Autodesk Fusion 360 part; units mm, degrees
(part 3 of 3)
  spline S37 degree 5 poles (-0.4472, -23.7562) (-0.4505, -23.7623) (-0.4571, -23.7746) (-0.4669, -23.793) (-0.4799, -23.8176) (-0.496, -23.8484) (-0.512, -23.8792) (-0.5278, -23.91) (-0.5434, -23.9408) (-0.5589, -23.9717) (-0.5742, -24.0026) (-0.5894, -24.0336) (-0.6044, -24.0645) (-0.6192, -24.0955) (-0.6339, -24.1265) (-0.6484, -24.1575) (-0.6627, -24.1886) (-0.6769, -24.2197) (-0.6909, -24.2508) (-0.7047, -24.2819) (-0.7183, -24.3131) (-0.7318, -24.3442) (-0.7451, -24.3754) (-0.7583, -24.4066) (-0.7712, -24.4379) (-0.784, -24.4691) (-0.7966, -24.5004) (-0.809, -24.5317) (-0.8213, -24.563) (-0.8333, -24.5943) (-0.8452, -24.6257) (-0.8569, -24.657) (-0.8684, -24.6884) (-0.8797, -24.7198) (-0.8908, -24.7512) (-0.9017, -24.7826) (-0.9124, -24.8141) (-0.923, -24.8455) (-0.9333, -24.877) (-0.9434, -24.9085) (-0.9533, -24.94) (-0.963, -24.9715) (-0.9725, -25.003) (-0.9818, -25.0346) (-0.9909, -25.0661) (-0.9997, -25.0977) (-1.0083, -25.1292) (-1.0168, -25.1608) (-1.0249, -25.1924) (-1.0329, -25.224) (-1.0406, -25.2556) (-1.048, -25.2872) (-1.0552, -25.3188) (-1.0622, -25.3504) (-1.0688, -25.382) (-1.0752, -25.4136) (-1.0814, -25.4452) (-1.0873, -25.4768) (-1.093, -25.5084) (-1.0984, -25.5401) (-1.1035, -25.5717) (-1.1081, -25.6033) (-1.1123, -25.6349) (-1.1161, -25.6665) (-1.1196, -25.6981) (-1.1227, -25.7297) (-1.1257, -25.7612) (-1.1284, -25.7928) (-1.1308, -25.8243) (-1.1327, -25.8558) (-1.1337, -25.8873) (-1.1335, -25.9124) (-1.1327, -25.9313) (-1.1319, -25.9438) (-1.1314, -25.9501) knots -1 -1 -1 -1 -1 -1 -0.98571429 -0.97142857 -0.95714286 -0.94285714 -0.92857143 -0.91428571 -0.9 -0.88571429 -0.87142857 -0.85714286 -0.84285714 -0.82857143 -0.81428571 -0.8 -0.78571429 -0.77142857 -0.75714286 -0.74285714 -0.72857143 -0.71428571 -0.7 -0.68571429 -0.67142857 -0.65714286 -0.64285714 -0.62857143 -0.61428571 -0.6 -0.58571429 -0.57142857 -0.55714286 -0.54285714 -0.52857143 -0.51428571 -0.5 -0.48571429 -0.47142857 -0.45714286 -0.44285714 -0.42857143 -0.41428571 -0.4 -0.38571429 -0.37142857 -0.35714286 -0.34285714 -0.32857143 -0.31428571 -0.3 -0.28571429 -0.27142857 -0.25714286 -0.24285714 -0.22857143 -0.21428571 -0.2 -0.18571429 -0.17142857 -0.15714286 -0.14285714 -0.12857143 -0.11428571 -0.1 -0.08571429 -0.07142857 -0.05714286 -0.04285714 -0.02857143 -0.01428571 0 0 0 0 0 0
  line L37 (-1.1314, -25.9501) -> (-1.0999, -26.3476)
  arc A75 (-1.3245, -26.6162) -> (-1.0999, -26.3476) centre (-1.3491, -26.3674) ccw
  arc A76 (-1.3245, -26.6162) -> (-2.1846, -26.7294) centre (0, -40) ccw
  arc A77 (-2.4711, -26.5282) -> (-2.1846, -26.7294) centre (-2.2252, -26.4827) ccw
  line L38 (-2.4711, -26.5282) -> (-2.5435, -26.136)
  spline S38 degree 5 poles (-2.5435, -26.136) (-2.5447, -26.1298) (-2.5471, -26.1175) (-2.5512, -26.0991) (-2.5576, -26.0747) (-2.5667, -26.0446) (-2.5766, -26.0146) (-2.5871, -25.9848) (-2.5979, -25.9551) (-2.609, -25.9253) (-2.6202, -25.8956) (-2.6317, -25.866) (-2.6435, -25.8365) (-2.6558, -25.807) (-2.6685, -25.7777) (-2.6815, -25.7485) (-2.6949, -25.7193) (-2.7086, -25.6903) (-2.7225, -25.6613) (-2.7367, -25.6323) (-2.751, -25.6034) (-2.7656, -25.5746) (-2.7805, -25.5459) (-2.7956, -25.5172) (-2.811, -25.4886) (-2.8266, -25.4601) (-2.8425, -25.4317) (-2.8586, -25.4033) (-2.8749, -25.375) (-2.8914, -25.3467) (-2.9081, -25.3185) (-2.925, -25.2904) (-2.9421, -25.2623) (-2.9594, -25.2343) (-2.977, -25.2064) (-2.9947, -25.1786) (-3.0126, -25.1508) (-3.0307, -25.123) (-3.0491, -25.0954) (-3.0675, -25.0678) (-3.0862, -25.0403) (-3.1051, -25.0128) (-3.1241, -24.9854) (-3.1434, -24.958) (-3.1628, -24.9308) (-3.1823, -24.9036) (-3.2021, -24.8764) (-3.222, -24.8494) (-3.2421, -24.8223) (-3.2624, -24.7954) (-3.2828, -24.7685) (-3.3034, -24.7417) (-3.3242, -24.715) (-3.3451, -24.6883) (-3.3662, -24.6617) (-3.3875, -24.6351) (-3.4089, -24.6086) (-3.4304, -24.5822) (-3.4522, -24.5558) (-3.4741, -24.5296) (-3.4961, -24.5033) (-3.5183, -24.4772) (-3.5406, -24.4511) (-3.5631, -24.4251) (-3.5858, -24.3991) (-3.6086, -24.3732) (-3.6315, -24.3474) (-3.6546, -24.3216) (-3.6779, -24.296) (-3.7012, -24.2703) (-3.7248, -24.2448) (-3.7437, -24.2244) (-3.758, -24.2092) (-3.7675, -24.199) (-3.7723, -24.1939) knots 0 0 0 0 0 0 0.01428571 0.02857143 0.04285714 0.05714286 0.07142857 0.08571429 0.1 0.11428571 0.12857143 0.14285714 0.15714286 0.17142857 0.18571429 0.2 0.21428571 0.22857143 0.24285714 0.25714286 0.27142857 0.28571429 0.3 0.31428571 0.32857143 0.34285714 0.35714286 0.37142857 0.38571429 0.4 0.41428571 0.42857143 0.44285714 0.45714286 0.47142857 0.48571429 0.5 0.51428571 0.52857143 0.54285714 0.55714286 0.57142857 0.58571429 0.6 0.61428571 0.62857143 0.64285714 0.65714286 0.67142857 0.68571429 0.7 0.71428571 0.72857143 0.74285714 0.75714286 0.77142857 0.78571429 0.8 0.81428571 0.82857143 0.84285714 0.85714286 0.87142857 0.88571429 0.9 0.91428571 0.92857143 0.94285714 0.95714286 0.97142857 0.98571429 1 1 1 1 1 1
  arc A78 (-3.7723, -24.1939) -> (-4.6361, -24.4254) centre (0, -40) ccw
  spline S39 degree 5 poles (-4.6361, -24.4254) (-4.6377, -24.4322) (-4.6409, -24.4457) (-4.6457, -24.4661) (-4.6519, -24.4932) (-4.6595, -24.5271) (-4.6669, -24.561) (-4.6742, -24.5948) (-4.6813, -24.6287) (-4.6883, -24.6625) (-4.6951, -24.6963) (-4.7017, -24.7301) (-4.7082, -24.7639) (-4.7145, -24.7977) (-4.7206, -24.8314) (-4.7266, -24.8652) (-4.7324, -24.8989) (-4.738, -24.9326) (-4.7435, -24.9662) (-4.7488, -24.9999) (-4.754, -25.0335) (-4.7589, -25.0671) (-4.7637, -25.1007) (-4.7683, -25.1342) (-4.7727, -25.1677) (-4.777, -25.2012) (-4.7811, -25.2347) (-4.785, -25.2681) (-4.7887, -25.3016) (-4.7922, -25.3349) (-4.7956, -25.3683) (-4.7987, -25.4016) (-4.8017, -25.4349) (-4.8045, -25.4681) (-4.8071, -25.5014) (-4.8095, -25.5345) (-4.8118, -25.5677) (-4.8138, -25.6008) (-4.8156, -25.6339) (-4.8172, -25.6669) (-4.8187, -25.6999) (-4.8199, -25.7328) (-4.8209, -25.7658) (-4.8217, -25.7986) (-4.8223, -25.8314) (-4.8227, -25.8642) (-4.8228, -25.8969) (-4.8228, -25.9296) (-4.8225, -25.9622) (-4.822, -25.9948) (-4.8213, -26.0273) (-4.8203, -26.0597) (-4.8191, -26.0921) (-4.8176, -26.1244) (-4.8158, -26.1567) (-4.8138, -26.1889) (-4.8116, -26.221) (-4.8092, -26.2531) (-4.8065, -26.2851) (-4.8035, -26.3171) (-4.8002, -26.3489) (-4.7965, -26.3806) (-4.7924, -26.4123) (-4.7879, -26.4438) (-4.783, -26.4752) (-4.7779, -26.5065) (-4.7726, -26.5377) (-4.7671, -26.5689) (-4.7613, -26.6) (-4.7549, -26.6309) (-4.7477, -26.6616) (-4.741, -26.6858) (-4.7354, -26.7038) (-4.7313, -26.7157) (-4.7292, -26.7217) knots -1 -1 -1 -1 -1 -1 -0.98571429 -0.97142857 -0.95714286 -0.94285714 -0.92857143 -0.91428571 -0.9 -0.88571429 -0.87142857 -0.85714286 -0.84285714 -0.82857143 -0.81428571 -0.8 -0.78571429 -0.77142857 -0.75714286 -0.74285714 -0.72857143 -0.71428571 -0.7 -0.68571429 -0.67142857 -0.65714286 -0.64285714 -0.62857143 -0.61428571 -0.6 -0.58571429 -0.57142857 -0.55714286 -0.54285714 -0.52857143 -0.51428571 -0.5 -0.48571429 -0.47142857 -0.45714286 -0.44285714 -0.42857143 -0.41428571 -0.4 -0.38571429 -0.37142857 -0.35714286 -0.34285714 -0.32857143 -0.31428571 -0.3 -0.28571429 -0.27142857 -0.25714286 -0.24285714 -0.22857143 -0.21428571 -0.2 -0.18571429 -0.17142857 -0.15714286 -0.14285714 -0.12857143 -0.11428571 -0.1 -0.08571429 -0.07142857 -0.05714286 -0.04285714 -0.02857143 -0.01428571 0 0 0 0 0 0
  line L39 (-4.7292, -26.7217) -> (-4.5959, -27.0975)
  arc A79 (-4.7433, -27.415) -> (-4.5959, -27.0975) centre (-4.8315, -27.1811) ccw
  arc A80 (-4.7433, -27.415) -> (-5.5449, -27.747) centre (0, -40) ccw
  arc A81 (-5.8737, -27.6268) -> (-5.5449, -27.747) centre (-5.648, -27.5193) ccw
  line L40 (-5.8737, -27.6268) -> (-6.0451, -27.2667)
  spline S40 degree 5 poles (-6.0451, -27.2667) (-6.0478, -27.261) (-6.0534, -27.2497) (-6.0621, -27.233) (-6.0745, -27.2112) (-6.0911, -27.1844) (-6.1085, -27.1581) (-6.1264, -27.132) (-6.1445, -27.106) (-6.1629, -27.0802) (-6.1814, -27.0544) (-6.2002, -27.0287) (-6.2193, -27.0033) (-6.2387, -26.978) (-6.2585, -26.953) (-6.2787, -26.9281) (-6.2992, -26.9034) (-6.3199, -26.8789) (-6.3409, -26.8545) (-6.362, -26.8302) (-6.3834, -26.806) (-6.405, -26.782) (-6.4268, -26.7581) (-6.4488, -26.7343) (-6.471, -26.7106) (-6.4935, -26.6871) (-6.5162, -26.6638) (-6.5391, -26.6405) (-6.5621, -26.6174) (-6.5854, -26.5943) (-6.6088, -26.5714) (-6.6324, -26.5486) (-6.6562, -26.526) (-6.6802, -26.5034) (-6.7044, -26.481) (-6.7287, -26.4587) (-6.7532, -26.4365) (-6.7779, -26.4144) (-6.8028, -26.3924) (-6.8278, -26.3705) (-6.8529, -26.3488) (-6.8783, -26.3271) (-6.9038, -26.3056) (-6.9294, -26.2842) (-6.9552, -26.2628) (-6.9812, -26.2416) (-7.0073, -26.2205) (-7.0335, -26.1995) (-7.0599, -26.1786) (-7.0865, -26.1578) (-7.1132, -26.1372) (-7.14, -26.1166) (-7.167, -26.0961) (-7.1941, -26.0758) (-7.2214, -26.0555) (-7.2488, -26.0354) (-7.2763, -26.0153) (-7.304, -25.9954) (-7.3318, -25.9756) (-7.3597, -25.9558) (-7.3878, -25.9362) (-7.416, -25.9167) (-7.4443, -25.8973) (-7.4728, -25.878) (-7.5014, -25.8588) (-7.5301, -25.8397) (-7.559, -25.8207) (-7.5879, -25.8018) (-7.617, -25.783) (-7.6463, -25.7643) (-7.6756, -25.7457) (-7.6992, -25.7309) (-7.7169, -25.7198) (-7.7287, -25.7125) (-7.7347, -25.7088) knots 0 0 0 0 0 0 0.01428571 0.02857143 0.04285714 0.05714286 0.07142857 0.08571429 0.1 0.11428571 0.12857143 0.14285714 0.15714286 0.17142857 0.18571429 0.2 0.21428571 0.22857143 0.24285714 0.25714286 0.27142857 0.28571429 0.3 0.31428571 0.32857143 0.34285714 0.35714286 0.37142857 0.38571429 0.4 0.41428571 0.42857143 0.44285714 0.45714286 0.47142857 0.48571429 0.5 0.51428571 0.52857143 0.54285714 0.55714286 0.57142857 0.58571429 0.6 0.61428571 0.62857143 0.64285714 0.65714286 0.67142857 0.68571429 0.7 0.71428571 0.72857143 0.74285714 0.75714286 0.77142857 0.78571429 0.8 0.81428571 0.82857143 0.84285714 0.85714286 0.87142857 0.88571429 0.9 0.91428571 0.92857143 0.94285714 0.95714286 0.97142857 0.98571429 1 1 1 1 1 1
  arc A82 (-7.7347, -25.7088) -> (-8.5092, -26.156) centre (0, -40) ccw
  spline S41 degree 5 poles (-8.5092, -26.156) (-8.509, -26.163) (-8.5085, -26.1769) (-8.5078, -26.1978) (-8.5068, -26.2256) (-8.5054, -26.2603) (-8.5038, -26.2949) (-8.5021, -26.3295) (-8.5002, -26.3641) (-8.4982, -26.3986) (-8.496, -26.433) (-8.4936, -26.4673) (-8.4911, -26.5017) (-8.4885, -26.5359) (-8.4857, -26.5701) (-8.4827, -26.6042) (-8.4796, -26.6383) (-8.4763, -26.6723) (-8.4729, -26.7062) (-8.4693, -26.7401) (-8.4656, -26.7739) (-8.4617, -26.8076) (-8.4576, -26.8413) (-8.4534, -26.8749) (-8.449, -26.9084) (-8.4444, -26.9419) (-8.4397, -26.9752) (-8.4348, -27.0086) (-8.4298, -27.0418) (-8.4245, -27.075) (-8.4191, -27.108) (-8.4136, -27.141) (-8.4078, -27.174) (-8.4019, -27.2068) (-8.3958, -27.2396) (-8.3896, -27.2722) (-8.3832, -27.3048) (-8.3765, -27.3373) (-8.3697, -27.3698) (-8.3628, -27.4021) (-8.3556, -27.4343) (-8.3483, -27.4665) (-8.3407, -27.4985) (-8.333, -27.5305) (-8.3251, -27.5623) (-8.3169, -27.5941) (-8.3086, -27.6257) (-8.3001, -27.6572) (-8.2914, -27.6887) (-8.2825, -27.72) (-8.2734, -27.7512) (-8.2641, -27.7823) (-8.2545, -27.8133) (-8.2447, -27.8441) (-8.2346, -27.8748) (-8.2244, -27.9054) (-8.2139, -27.9359) (-8.2032, -27.9662) (-8.1924, -27.9965) (-8.1812, -28.0265) (-8.1698, -28.0564) (-8.158, -28.0861) (-8.1459, -28.1156) (-8.1334, -28.1449) (-8.1205, -28.174) (-8.1075, -28.2029) (-8.0943, -28.2317) (-8.0808, -28.2604) (-8.0672, -28.2889) (-8.0531, -28.3171) (-8.0382, -28.3449) (-8.0255, -28.3666) (-8.0154, -28.3825) (-8.0083, -28.3929) (-8.0048, -28.3981) knots -1 -1 -1 -1 -1 -1 -0.98571429 -0.97142857 -0.95714286 -0.94285714 -0.92857143 -0.91428571 -0.9 -0.88571429 -0.87142857 -0.85714286 -0.84285714 -0.82857143 -0.81428571 -0.8 -0.78571429 -0.77142857 -0.75714286 -0.74285714 -0.72857143 -0.71428571 -0.7 -0.68571429 -0.67142857 -0.65714286 -0.64285714 -0.62857143 -0.61428571 -0.6 -0.58571429 -0.57142857 -0.55714286 -0.54285714 -0.52857143 -0.51428571 -0.5 -0.48571429 -0.47142857 -0.45714286 -0.44285714 -0.42857143 -0.41428571 -0.4 -0.38571429 -0.37142857 -0.35714286 -0.34285714 -0.32857143 -0.31428571 -0.3 -0.28571429 -0.27142857 -0.25714286 -0.24285714 -0.22857143 -0.21428571 -0.2 -0.18571429 -0.17142857 -0.15714286 -0.14285714 -0.12857143 -0.11428571 -0.1 -0.08571429 -0.07142857 -0.05714286 -0.04285714 -0.02857143 -0.01428571 0 0 0 0 0 0
  line L41 (-8.0048, -28.3981) -> (-7.7787, -28.7266)
  arc A83 (-7.8389, -29.0715) -> (-7.7787, -28.7266) centre (-7.9847, -28.8684) ccw
  arc A84 (-7.8389, -29.0715) -> (-8.5272, -29.5997) centre (0, -40) ccw
  arc A85 (-8.876, -29.5686) -> (-8.5272, -29.5997) centre (-8.6858, -29.4063) ccw
  line L42 (-8.876, -29.5686) -> (-9.1348, -29.2652)
  spline S42 degree 5 poles (-9.1348, -29.2652) (-9.1388, -29.2604) (-9.1471, -29.2509) (-9.1599, -29.2371) (-9.1775, -29.2191) (-9.2005, -29.1976) (-9.2241, -29.1766) (-9.2481, -29.1561) (-9.2724, -29.1357) (-9.2968, -29.1155) (-9.3213, -29.0954) (-9.3461, -29.0755) (-9.3711, -29.0558) (-9.3965, -29.0364) (-9.4221, -29.0174) (-9.448, -28.9986) (-9.4742, -28.98) (-9.5006, -28.9617) (-9.5271, -28.9435) (-9.5539, -28.9256) (-9.5807, -28.9077) (-9.6078, -28.8901) (-9.635, -28.8726) (-9.6625, -28.8554) (-9.6901, -28.8383) (-9.7179, -28.8214) (-9.7458, -28.8047) (-9.7739, -28.7881) (-9.8022, -28.7718) (-9.8306, -28.7556) (-9.8592, -28.7395) (-9.8879, -28.7236) (-9.9168, -28.7079) (-9.9458, -28.6923) (-9.9749, -28.6769) (-10.0042, -28.6616) (-10.0336, -28.6465) (-10.0632, -28.6315) (-10.0929, -28.6167) (-10.1227, -28.6021) (-10.1526, -28.5876) (-10.1827, -28.5732) (-10.2129, -28.559) (-10.2432, -28.545) (-10.2736, -28.5311) (-10.3042, -28.5173) (-10.3349, -28.5037) (-10.3657, -28.4902) (-10.3966, -28.4768) (-10.4276, -28.4636) (-10.4588, -28.4506) (-10.49, -28.4376) (-10.5214, -28.4249) (-10.5528, -28.4122) (-10.5844, -28.3997) (-10.6161, -28.3873) (-10.6479, -28.3751) (-10.6798, -28.363) (-10.7118, -28.3511) (-10.7438, -28.3392) (-10.776, -28.3275) (-10.8083, -28.316) (-10.8407, -28.3046) (-10.8732, -28.2933) (-10.9058, -28.2821) (-10.9385, -28.2711) (-10.9713, -28.2602) (-11.0042, -28.2495) (-11.0371, -28.2388) (-11.0702, -28.2283) (-11.1033, -28.218) (-11.1299, -28.2098) (-11.1499, -28.2037) (-11.1633, -28.1997) (-11.1699, -28.1977) knots 0 0 0 0 0 0 0.01428571 0.02857143 0.04285714 0.05714286 0.07142857 0.08571429 0.1 0.11428571 0.12857143 0.14285714 0.15714286 0.17142857 0.18571429 0.2 0.21428571 0.22857143 0.24285714 0.25714286 0.27142857 0.28571429 0.3 0.31428571 0.32857143 0.34285714 0.35714286 0.37142857 0.38571429 0.4 0.41428571 0.42857143 0.44285714 0.45714286 0.47142857 0.48571429 0.5 0.51428571 0.52857143 0.54285714 0.55714286 0.57142857 0.58571429 0.6 0.61428571 0.62857143 0.64285714 0.65714286 0.67142857 0.68571429 0.7 0.71428571 0.72857143 0.74285714 0.75714286 0.77142857 0.78571429 0.8 0.81428571 0.82857143 0.84285714 0.85714286 0.87142857 0.88571429 0.9 0.91428571 0.92857143 0.94285714 0.95714286 0.97142857 0.98571429 1 1 1 1 1 1
  arc A86 (-11.1699, -28.1977) -> (-11.8023, -28.8301) centre (0, -40) ccw
  spline S43 degree 5 poles (-11.8023, -28.8301) (-11.8003, -28.8367) (-11.7963, -28.8501) (-11.7902, -28.8701) (-11.782, -28.8967) (-11.7717, -28.9298) (-11.7612, -28.9629) (-11.7505, -28.9958) (-11.7398, -29.0287) (-11.7289, -29.0615) (-11.7179, -29.0942) (-11.7067, -29.1268) (-11.6954, -29.1593) (-11.684, -29.1917) (-11.6725, -29.224) (-11.6608, -29.2562) (-11.6489, -29.2882) (-11.637, -29.3202) (-11.6249, -29.3521) (-11.6127, -29.3839) (-11.6003, -29.4156) (-11.5878, -29.4472) (-11.5751, -29.4786) (-11.5624, -29.51) (-11.5494, -29.5412) (-11.5364, -29.5724) (-11.5232, -29.6034) (-11.5098, -29.6343) (-11.4963, -29.6651) (-11.4827, -29.6958) (-11.4689, -29.7264) (-11.455, -29.7568) (-11.441, -29.7871) (-11.4268, -29.8173) (-11.4124, -29.8474) (-11.3979, -29.8773) (-11.3833, -29.9071) (-11.3685, -29.9368) (-11.3535, -29.9664) (-11.3384, -29.9958) (-11.3231, -30.0251) (-11.3077, -30.0542) (-11.2921, -30.0832) (-11.2764, -30.1121) (-11.2605, -30.1408) (-11.2444, -30.1694) (-11.2282, -30.1978) (-11.2119, -30.2261) (-11.1953, -30.2542) (-11.1786, -30.2821) (-11.1617, -30.3099) (-11.1446, -30.3375) (-11.1274, -30.365) (-11.1099, -30.3922) (-11.0923, -30.4193) (-11.0744, -30.4461) (-11.0565, -30.4729) (-11.0383, -30.4994) (-11.02, -30.5258) (-11.0014, -30.552) (-10.9826, -30.5779) (-10.9636, -30.6035) (-10.9442, -30.6289) (-10.9245, -30.6539) (-10.9046, -30.6787) (-10.8845, -30.7032) (-10.8643, -30.7276) (-10.8439, -30.7519) (-10.8234, -30.7759) (-10.8024, -30.7995) (-10.7809, -30.8225) (-10.7629, -30.8401) (-10.7491, -30.8529) (-10.7396, -30.8612) (-10.7348, -30.8652) knots -1 -1 -1 -1 -1 -1 -0.98571429 -0.97142857 -0.95714286 -0.94285714 -0.92857143 -0.91428571 -0.9 -0.88571429 -0.87142857 -0.85714286 -0.84285714 -0.82857143 -0.81428571 -0.8 -0.78571429 -0.77142857 -0.75714286 -0.74285714 -0.72857143 -0.71428571 -0.7 -0.68571429 -0.67142857 -0.65714286 -0.64285714 -0.62857143 -0.61428571 -0.6 -0.58571429 -0.57142857 -0.55714286 -0.54285714 -0.52857143 -0.51428571 -0.5 -0.48571429 -0.47142857 -0.45714286 -0.44285714 -0.42857143 -0.41428571 -0.4 -0.38571429 -0.37142857 -0.35714286 -0.34285714 -0.32857143 -0.31428571 -0.3 -0.28571429 -0.27142857 -0.25714286 -0.24285714 -0.22857143 -0.21428571 -0.2 -0.18571429 -0.17142857 -0.15714286 -0.14285714 -0.12857143 -0.11428571 -0.1 -0.08571429 -0.07142857 -0.05714286 -0.04285714 -0.02857143 -0.01428571 0 0 0 0 0 0
  line L43 (-10.7348, -30.8652) -> (-10.4314, -31.124)
  arc A87 (-10.4003, -31.4728) -> (-10.4314, -31.124) centre (-10.5937, -31.3142) ccw
  arc A88 (-10.4003, -31.4728) -> (-10.9285, -32.1611) centre (0, -40) ccw
  arc A89 (-11.2734, -32.2213) -> (-10.9285, -32.1611) centre (-11.1316, -32.0153) ccw
  line L44 (-11.2734, -32.2213) -> (-11.6019, -31.9952)
  spline S44 degree 5 poles (-11.6019, -31.9952) (-11.6071, -31.9917) (-11.6175, -31.9846) (-11.6334, -31.9745) (-11.6551, -31.9618) (-11.6829, -31.9469) (-11.7111, -31.9328) (-11.7396, -31.9192) (-11.7683, -31.9057) (-11.7971, -31.8925) (-11.826, -31.8795) (-11.8551, -31.8666) (-11.8844, -31.8541) (-11.9139, -31.842) (-11.9436, -31.8302) (-11.9735, -31.8188) (-12.0035, -31.8076) (-12.0338, -31.7968) (-12.0641, -31.7861) (-12.0946, -31.7756) (-12.1252, -31.7654) (-12.1559, -31.7553) (-12.1867, -31.7455) (-12.2177, -31.7359) (-12.2488, -31.7266) (-12.28, -31.7175) (-12.3113, -31.7086) (-12.3428, -31.6999) (-12.3743, -31.6914) (-12.4059, -31.6831) (-12.4377, -31.6749) (-12.4695, -31.667) (-12.5015, -31.6593) (-12.5335, -31.6517) (-12.5657, -31.6444) (-12.5979, -31.6372) (-12.6302, -31.6303) (-12.6627, -31.6235) (-12.6952, -31.6168) (-12.7278, -31.6104) (-12.7604, -31.6042) (-12.7932, -31.5981) (-12.826, -31.5922) (-12.859, -31.5864) (-12.892, -31.5809) (-12.925, -31.5755) (-12.9582, -31.5702) (-12.9914, -31.5652) (-13.0248, -31.5603) (-13.0581, -31.5556) (-13.0916, -31.551) (-13.1251, -31.5466) (-13.1587, -31.5424) (-13.1924, -31.5383) (-13.2261, -31.5344) (-13.2599, -31.5307) (-13.2938, -31.5271) (-13.3277, -31.5237) (-13.3617, -31.5204) (-13.3958, -31.5173) (-13.4299, -31.5143) (-13.4641, -31.5115) (-13.4983, -31.5089) (-13.5327, -31.5064) (-13.567, -31.504) (-13.6014, -31.5018) (-13.6359, -31.4998) (-13.6705, -31.4979) (-13.7051, -31.4962) (-13.7397, -31.4946) (-13.7744, -31.4932) (-13.8022, -31.4922) (-13.8231, -31.4915) (-13.837, -31.491) (-13.844, -31.4908) knots 0 0 0 0 0 0 0.01428571 0.02857143 0.04285714 0.05714286 0.07142857 0.08571429 0.1 0.11428571 0.12857143 0.14285714 0.15714286 0.17142857 0.18571429 0.2 0.21428571 0.22857143 0.24285714 0.25714286 0.27142857 0.28571429 0.3 0.31428571 0.32857143 0.34285714 0.35714286 0.37142857 0.38571429 0.4 0.41428571 0.42857143 0.44285714 0.45714286 0.47142857 0.48571429 0.5 0.51428571 0.52857143 0.54285714 0.55714286 0.57142857 0.58571429 0.6 0.61428571 0.62857143 0.64285714 0.65714286 0.67142857 0.68571429 0.7 0.71428571 0.72857143 0.74285714 0.75714286 0.77142857 0.78571429 0.8 0.81428571 0.82857143 0.84285714 0.85714286 0.87142857 0.88571429 0.9 0.91428571 0.92857143 0.94285714 0.95714286 0.97142857 0.98571429 1 1 1 1 1 1
  arc A90 (-13.844, -31.4908) -> (-14.2912, -32.2653) centre (0, -40) ccw
  spline S45 degree 5 poles (-14.2912, -32.2653) (-14.2875, -32.2713) (-14.2802, -32.2831) (-14.2691, -32.3008) (-14.2543, -32.3244) (-14.2357, -32.3537) (-14.217, -32.383) (-14.1982, -32.4121) (-14.1793, -32.441) (-14.1603, -32.4699) (-14.1412, -32.4986) (-14.122, -32.5272) (-14.1027, -32.5557) (-14.0833, -32.584) (-14.0638, -32.6122) (-14.0442, -32.6403) (-14.0244, -32.6682) (-14.0046, -32.696) (-13.9847, -32.7237) (-13.9646, -32.7512) (-13.9445, -32.7786) (-13.9242, -32.8059) (-13.9039, -32.833) (-13.8834, -32.86) (-13.8628, -32.8868) (-13.8422, -32.9135) (-13.8214, -32.9401) (-13.8005, -32.9665) (-13.7795, -32.9927) (-13.7584, -33.0188) (-13.7372, -33.0448) (-13.7158, -33.0706) (-13.6944, -33.0962) (-13.6729, -33.1217) (-13.6512, -33.1471) (-13.6295, -33.1722) (-13.6076, -33.1972) (-13.5856, -33.2221) (-13.5635, -33.2468) (-13.5413, -33.2713) (-13.519, -33.2956) (-13.4966, -33.3198) (-13.474, -33.3438) (-13.4514, -33.3676) (-13.4286, -33.3912) (-13.4057, -33.4146) (-13.3826, -33.4379) (-13.3595, -33.4609) (-13.3362, -33.4838) (-13.3129, -33.5065) (-13.2894, -33.529) (-13.2657, -33.5512) (-13.2419, -33.5732) (-13.218, -33.595) (-13.194, -33.6166) (-13.1698, -33.638) (-13.1455, -33.6591) (-13.1211, -33.6801) (-13.0966, -33.7008) (-13.0719, -33.7213) (-13.047, -33.7415) (-13.022, -33.7613) (-12.9967, -33.7807) (-12.9713, -33.7998) (-12.9456, -33.8186) (-12.9198, -33.8371) (-12.894, -33.8555) (-12.868, -33.8736) (-12.8419, -33.8915) (-12.8156, -33.9089) (-12.7888, -33.9255) (-12.767, -33.9379) (-12.7503, -33.9466) (-12.739, -33.9522) (-12.7333, -33.9549) knots -1 -1 -1 -1 -1 -1 -0.98571429 -0.97142857 -0.95714286 -0.94285714 -0.92857143 -0.91428571 -0.9 -0.88571429 -0.87142857 -0.85714286 -0.84285714 -0.82857143 -0.81428571 -0.8 -0.78571429 -0.77142857 -0.75714286 -0.74285714 -0.72857143 -0.71428571 -0.7 -0.68571429 -0.67142857 -0.65714286 -0.64285714 -0.62857143 -0.61428571 -0.6 -0.58571429 -0.57142857 -0.55714286 -0.54285714 -0.52857143 -0.51428571 -0.5 -0.48571429 -0.47142857 -0.45714286 -0.44285714 -0.42857143 -0.41428571 -0.4 -0.38571429 -0.37142857 -0.35714286 -0.34285714 -0.32857143 -0.31428571 -0.3 -0.28571429 -0.27142857 -0.25714286 -0.24285714 -0.22857143 -0.21428571 -0.2 -0.18571429 -0.17142857 -0.15714286 -0.14285714 -0.12857143 -0.11428571 -0.1 -0.08571429 -0.07142857 -0.05714286 -0.04285714 -0.02857143 -0.01428571 0 0 0 0 0 0
  line L45 (-12.7333, -33.9549) -> (-12.3732, -34.1263)
  arc A91 (-12.253, -34.4551) -> (-12.3732, -34.1263) centre (-12.4807, -34.352) ccw
  arc A92 (-12.253, -34.4551) -> (-12.585, -35.2567) centre (0, -40) ccw
  arc A93 (-12.9025, -35.4041) -> (-12.585, -35.2567) centre (-12.8189, -35.1685) ccw
  line L46 (-12.9025, -35.4041) -> (-13.2783, -35.2708)
  spline S46 degree 5 poles (-13.2783, -35.2708) (-13.2843, -35.2687) (-13.2962, -35.2646) (-13.3142, -35.259) (-13.3384, -35.2523) (-13.3691, -35.2451) (-13.4, -35.2387) (-13.4311, -35.2329) (-13.4623, -35.2274) (-13.4935, -35.2221) (-13.5248, -35.217) (-13.5562, -35.2121) (-13.5877, -35.2076) (-13.6194, -35.2035) (-13.6511, -35.1998) (-13.6829, -35.1965) (-13.7149, -35.1935) (-13.7469, -35.1908) (-13.779, -35.1884) (-13.8111, -35.1862) (-13.8433, -35.1842) (-13.8756, -35.1824) (-13.9079, -35.1809) (-13.9403, -35.1797) (-13.9727, -35.1787) (-14.0052, -35.178) (-14.0378, -35.1775) (-14.0704, -35.1772) (-14.1031, -35.1772) (-14.1358, -35.1773) (-14.1686, -35.1777) (-14.2014, -35.1783) (-14.2342, -35.1791) (-14.2672, -35.1801) (-14.3001, -35.1813) (-14.3331, -35.1828) (-14.3661, -35.1844) (-14.3992, -35.1862) (-14.4323, -35.1882) (-14.4655, -35.1905) (-14.4986, -35.1929) (-14.5319, -35.1955) (-14.5651, -35.1983) (-14.5984, -35.2013) (-14.6317, -35.2044) (-14.6651, -35.2078) (-14.6984, -35.2113) (-14.7319, -35.215) (-14.7653, -35.2189) (-14.7988, -35.223) (-14.8323, -35.2273) (-14.8658, -35.2317) (-14.8993, -35.2363) (-14.9329, -35.2411) (-14.9665, -35.246) (-15.0001, -35.2512) (-15.0338, -35.2565) (-15.0674, -35.262) (-15.1011, -35.2676) (-15.1348, -35.2734) (-15.1686, -35.2794) (-15.2023, -35.2855) (-15.2361, -35.2918) (-15.2699, -35.2983) (-15.3037, -35.3049) (-15.3375, -35.3117) (-15.3713, -35.3187) (-15.4052, -35.3258) (-15.439, -35.3331) (-15.4729, -35.3405) (-15.5068, -35.3481) (-15.5339, -35.3543) (-15.5543, -35.3591) (-15.5678, -35.3623) (-15.5746, -35.3639) knots 0 0 0 0 0 0 0.01428571 0.02857143 0.04285714 0.05714286 0.07142857 0.08571429 0.1 0.11428571 0.12857143 0.14285714 0.15714286 0.17142857 0.18571429 0.2 0.21428571 0.22857143 0.24285714 0.25714286 0.27142857 0.28571429 0.3 0.31428571 0.32857143 0.34285714 0.35714286 0.37142857 0.38571429 0.4 0.41428571 0.42857143 0.44285714 0.45714286 0.47142857 0.48571429 0.5 0.51428571 0.52857143 0.54285714 0.55714286 0.57142857 0.58571429 0.6 0.61428571 0.62857143 0.64285714 0.65714286 0.67142857 0.68571429 0.7 0.71428571 0.72857143 0.74285714 0.75714286 0.77142857 0.78571429 0.8 0.81428571 0.82857143 0.84285714 0.85714286 0.87142857 0.88571429 0.9 0.91428571 0.92857143 0.94285714 0.95714286 0.97142857 0.98571429 1 1 1 1 1 1
  arc A94 (-15.5746, -35.3639) -> (-15.8061, -36.2277) centre (0, -40) ccw
  spline S47 degree 5 poles (-15.8061, -36.2277) (-15.801, -36.2325) (-15.7908, -36.242) (-15.7756, -36.2563) (-15.7552, -36.2752) (-15.7297, -36.2988) (-15.704, -36.3221) (-15.6784, -36.3454) (-15.6526, -36.3685) (-15.6268, -36.3914) (-15.6009, -36.4142) (-15.5749, -36.4369) (-15.5489, -36.4594) (-15.5228, -36.4817) (-15.4967, -36.5039) (-15.4704, -36.5259) (-15.4442, -36.5478) (-15.4178, -36.5696) (-15.3914, -36.5911) (-15.3649, -36.6125) (-15.3383, -36.6338) (-15.3117, -36.6549) (-15.285, -36.6758) (-15.2583, -36.6966) (-15.2315, -36.7172) (-15.2046, -36.7376) (-15.1777, -36.7579) (-15.1506, -36.778) (-15.1236, -36.7979) (-15.0964, -36.8177) (-15.0692, -36.8372) (-15.042, -36.8566) (-15.0146, -36.8759) (-14.9872, -36.8949) (-14.9597, -36.9138) (-14.9322, -36.9325) (-14.9046, -36.9509) (-14.877, -36.9693) (-14.8492, -36.9874) (-14.8214, -37.0053) (-14.7936, -37.023) (-14.7657, -37.0406) (-14.7377, -37.0579) (-14.7096, -37.075) (-14.6815, -37.0919) (-14.6533, -37.1086) (-14.625, -37.1251) (-14.5967, -37.1414) (-14.5683, -37.1575) (-14.5399, -37.1734) (-14.5114, -37.189) (-14.4828, -37.2044) (-14.4541, -37.2195) (-14.4254, -37.2344) (-14.3966, -37.249) (-14.3677, -37.2633) (-14.3387, -37.2775) (-14.3097, -37.2914) (-14.2807, -37.3051) (-14.2515, -37.3185) (-14.2223, -37.3315) (-14.193, -37.3442) (-14.1635, -37.3565) (-14.134, -37.3683) (-14.1044, -37.3798) (-14.0747, -37.391) (-14.0449, -37.4021) (-14.0152, -37.4129) (-13.9854, -37.4234) (-13.9554, -37.4333) (-13.9253, -37.4424) (-13.9009, -37.4488) (-13.8825, -37.4529) (-13.8702, -37.4553) (-13.864, -37.4565) knots -1 -1 -1 -1 -1 -1 -0.98571429 -0.97142857 -0.95714286 -0.94285714 -0.92857143 -0.91428571 -0.9 -0.88571429 -0.87142857 -0.85714286 -0.84285714 -0.82857143 -0.81428571 -0.8 -0.78571429 -0.77142857 -0.75714286 -0.74285714 -0.72857143 -0.71428571 -0.7 -0.68571429 -0.67142857 -0.65714286 -0.64285714 -0.62857143 -0.61428571 -0.6 -0.58571429 -0.57142857 -0.55714286 -0.54285714 -0.52857143 -0.51428571 -0.5 -0.48571429 -0.47142857 -0.45714286 -0.44285714 -0.42857143 -0.41428571 -0.4 -0.38571429 -0.37142857 -0.35714286 -0.34285714 -0.32857143 -0.31428571 -0.3 -0.28571429 -0.27142857 -0.25714286 -0.24285714 -0.22857143 -0.21428571 -0.2 -0.18571429 -0.17142857 -0.15714286 -0.14285714 -0.12857143 -0.11428571 -0.1 -0.08571429 -0.07142857 -0.05714286 -0.04285714 -0.02857143 -0.01428571 0 0 0 0 0 0
  line L47 (-13.864, -37.4565) -> (-13.4718, -37.5289)
  arc A95 (-13.2706, -37.8154) -> (-13.4718, -37.5289) centre (-13.5173, -37.7748) ccw
  circle A96 centre (0, -40) radius 5.5
  dimension "d9" = 11
  constraint concentric A0 A96
  measures "d9" diameter of A96
extrude "Extrude1'" cut sketch "Sketch2 (2)" against normal blind 10 contours A96 bodies 2
thread "Thread1" "ISO Metric profile 11.0 M11x1.5 M11x1.5 6H" major diameter 11.1933 minor diameter 9.5262 pitch 1.5 angle 60 modelled right hand crest width 0.4125 on face at (-5.4932, 40.2742, 3.3333) crest through (-4.7631, 40, 9.625) on bodies 2
component "Spur Gear (24 teeth)" placed x (1, 0, 0) y (0, 1, 0) z (0, 0, 1) at (0, 0, 0)
